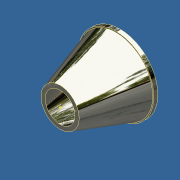
# Autodesk Inventor part: Parabol
Saved by Autodesk Inventor 2018.2 (Build 222227000, 227)
## iProperties
Created: 2018-10-30
Part Number: Parabol
Material: 1.4301 X 5 CrNi 18 10
Document SubType Name: Modeling
Designer: N.Grubert
Density: 8 g/cm^3
Appearance: Silber
Author: N.Grubert
Fläche: 0 cm²
Gewicht: 0 g
Material: geeigneten Werkstoff auswählen !
Dateiname: P:\INVENTOR\Inventor 2018\Templates\ILT\Norm.ipt
Bez_eng: bolt
Bez_french: boulon
Autodesk Inventor part; units mm, degrees
ref_plane "YZ Plane" through (0, 0, 0) normal (1, 0, 0) x (0, 1, 0)
ref_plane "XZ Plane" through (0, 0, 0) normal (0, 1, 0) x (-1, 0, 0)
ref_plane "XY Plane" through (0, 0, 0) normal (0, 0, 1) x (1, 0, 0)
sketch "Skizze4" plane through (0, 0, 0) normal (0, 0, 1) x (1, 0, 0)
  line L0 (0, -3) -> (0, 18) projected
  line L1 (-11.4593, 0) -> (1.9099, 0) construction
  line L2 (-9.5, 15) -> (-8.5, 15)
  line L3 (-8.5, 15) -> (-3.7271, 0)
  line L4 (-9.2312, 14) -> (-4.7765, 0)
  line L5 (-4.7765, 0) -> (-3.7271, 0)
  line L6 (-9.5, 15) -> (-8.4246, 15)
  line L7 (-9.2312, 14) -> (-9.5, 14)
  line L8 (-9.5, 14) -> (-9.5, 15)
  line L9 (-4.7765, 0) -> (-9.5494, 15) construction
  point P0 (0, 0)
  dimension "d4" = 9.553
  dimension "d5" = 19
  dimension "d6" = 1
  dimension "d8" = 15
  dimension "d11" = 1
  dimension "d12" = 1
  constraints: 16 end point, 4 point on line, 2 horizontal, 2 parallel, 1 collinear, 1 perpendicular
  measures "d4" diameter of L4.end L0
  measures "d5" diameter of L2.start L0
  measures "d6" distance between parallel lines of L3 L4
  measures "d8" distance between parallel lines of L2 L1
  measures "d11" distance of L2.start L2.end
  measures "d12" distance between parallel lines of L2 L7
revolve "Umdrehung1" add sketch "Skizze4" angle 360 about axis through (0, -10, 0) along (0, 1, 0)
